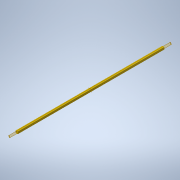
# Autodesk Inventor part: podest duzy profil 1
Saved by Autodesk Inventor 2021 (Build 250183000, 183)
## iProperties
Created: 2024-04-08
Part Number: podest duzy profil 1
Material: Steel
Document SubType Name: Modeling
Designer: Michal
Density: 7.85 g/cm^3
Appearance: Glossy - Gold
Author: Michal
Autodesk Inventor part; units mm, degrees
ref_plane "YZ Plane" through (0, 0, 0) normal (1, 0, 0) x (0, 1, 0)
ref_plane "XZ Plane" through (0, 0, 0) normal (0, 1, 0) x (-1, 0, 0)
ref_plane "XY Plane" through (0, 0, 0) normal (0, 0, 1) x (1, 0, 0)
sketch "Sketch1" plane through (0, 0, 0) normal (0, 1, 0) x (-1, 0, 0)
  line L0 (-12, 14) -> (12, 14) construction
  line L1 (14, 12) -> (14, -12) construction
  line L2 (12, -14) -> (-12, -14) construction
  line L3 (-14, -12) -> (-14, 12) construction
  line L4 (-14, 14) -> (14, -14) construction
  line L5 (14, 14) -> (-14, -14) construction
  arc A0 (14, 12) -> (12, 14) centre (12, 12) ccw construction
  arc A1 (12, -14) -> (14, -12) centre (12, -12) ccw construction
  arc A2 (-14, -12) -> (-12, -14) centre (-12, -12) ccw construction
  arc A3 (-12, 14) -> (-14, 12) centre (-12, 12) ccw construction
  line L6 (-12, -15) -> (12, -15)
  arc A4 (12, -15) -> (15, -12) centre (12, -12) ccw
  line L7 (15, -12) -> (15, 12)
  arc A5 (15, 12) -> (12, 15) centre (12, 12) ccw
  line L8 (12, 15) -> (-12, 15)
  arc A6 (-12, 15) -> (-15, 12) centre (-12, 12) ccw
  line L9 (-15, 12) -> (-15, -12)
  arc A7 (-15, -12) -> (-12, -15) centre (-12, -12) ccw
  line L10 (13, -12) -> (13, 12)
  arc A8 (13, 12) -> (12, 13) centre (12, 12) ccw
  line L11 (12, 13) -> (-12, 13)
  arc A9 (-12, 13) -> (-13, 12) centre (-12, 12) ccw
  line L12 (-13, 12) -> (-13, -12)
  arc A10 (-13, -12) -> (-12, -13) centre (-12, -12) ccw
  line L13 (-12, -13) -> (12, -13)
  arc A11 (12, -13) -> (13, -12) centre (12, -12) ccw
  point P0 (0, 0)
  point P1 (0, 0)
  point P2 (0, 0)
  dimension "d10" = 2
  dimension "depth" = 30
  dimension "width" = 30
  dimension "thickness" = 2
  constraints: 28 end point, 24 point on circle, 12 centre point, 8 point on line, 8 tangent, 6 parallel, 3 equal radius, 3 midpoint, 3 perpendicular, 1 coincident, 1 horizontal, 15 other
  measures "d10" radius of A0
  measures "depth" distance between parallel lines of L6 L8
  measures "width" distance between parallel lines of L9 L7
  measures "thickness" distance between parallel lines of L10 L7
extrude "Extrusion1" add sketch "Sketch1" along normal blind 2000
ref_plane "Work Plane1" through (0, 1000, 0) normal (0, -1, 0) x (1, 0, 0)
sketch "Sketch3" plane through (12, 0, -15) normal (0, 0, -1) x (-1, 0, 0)
  line L0 (12, -400) -> (12, 2400) construction
  circle A0 centre (-3, 1000) radius 985
  point P0 (12, 0)
  dimension "d29" = 1970
  dimension "d31" = 1000
  dimension "d34" = 15
  constraints: 1 centre point
  measures "d29" diameter of A0
  measures "d31" vertical distance of point (12, 0) A0.centre
  measures "d34" distance from line of A0.centre L0
extrude "Extrusion2" cut sketch "Sketch3" against normal through all keep common part
sketch "Sketch4" plane through (15, 15, 12) normal (1, 0, 0) x (0, 0, -1)
  line L0 (33.0025, 985) -> (-9.0025, 985) construction
  line L1 (12, -412.0004) -> (12, 2367.0022) projected
  point P0 (12, -15)
  point P1 (12, 235)
  point P2 (12, 985)
  point P3 (12, 1735)
  point P4 (12, 735)
  point P5 (12, 1235)
  dimension "d35" = 1500
  dimension "d36" = 500
  constraints: 3 point on line, 2 symmetric about line
  measures "d35" distance of point (12, 1735) point (12, 235)
  measures "d36" distance of point (12, 1235) point (12, 735)
hole "Hole2" at (15, 250, 0) at (15, 1750, 0) at (15, 750, 0) at (15, 1250, 0) direction (-1, 0, 0) diameter 8 depth 40 tip angle 118
equation "\"d10\" = thickness"
body "Solid1"
